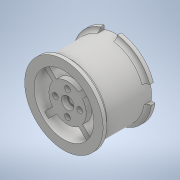
# Autodesk Inventor part: Wheel
Saved by Autodesk Inventor 2020 (Build 240168000, 168)
## iProperties
Created: 2019-03-25
Part Number: Wheel
Material: Типовые
Document SubType Name: Modeling
Designer: cosko
Density: 1 g/cm^3
Appearance: По умолчанию
Mass: 16.7421 g
Surface Area: 120.92 cm^2
Volume: 16.7421 cm^3
Author: cosko
Autodesk Inventor part; units mm, degrees
ref_plane "YZ Plane" through (0, 0, 0) normal (1, 0, 0) x (0, 1, 0)
ref_plane "XZ Plane" through (0, 0, 0) normal (0, 1, 0) x (-1, 0, 0)
ref_plane "XY Plane" through (0, 0, 0) normal (0, 0, 1) x (1, 0, 0)
sketch "Эскиз1" plane through (0, 0, 0) normal (0, 0, 1) x (1, 0, 0)
  line L0 (0, 0) -> (16, 0) construction
  line L1 (16, 0) -> (16, 12) construction
  line L2 (16, 12) -> (16, -16)
  line L3 (16, 12) -> (21, 12)
  line L4 (21, 12) -> (21, -16)
  line L5 (21, -16) -> (16, -16)
  line L6 (16, -16) -> (16, 12)
  line L7 (21, 12) -> (16, 12) construction
  line L8 (16, 12) -> (16, 10) construction
  line L9 (21, 10) -> (21, 10) construction
  line L10 (21, 10) -> (21, 12) construction
  line L11 (21, -16) -> (16, -16) construction
  line L12 (16, -16) -> (16, -14) construction
  line L13 (16, -14) -> (21, -14) construction
  line L14 (21, -14) -> (21, -16) construction
  line L15 (21, -14) -> (21, -14)
  line L16 (19, -12) -> (19, 8)
  line L17 (21, 6) -> (21, -14)
  arc A0 (21, 10) -> (19, 8) centre (21, 8) ccw
  arc A1 (19, -12) -> (21, -14) centre (21, -12) ccw
  arc A2 (21, 10) -> (19, 8) centre (21, 8) ccw
  line L18 (19, 8) -> (19, -12)
  arc A3 (19, -12) -> (21, -14) centre (21, -12) ccw
  line L19 (21, -14) -> (21, 10)
  line L20 (0, 0) -> (0, 12)
  dimension "d0" = 16
  dimension "d1" = 12
  dimension "d2" = 28
  dimension "d3" = 5
  dimension "d4" = 2
  dimension "d7" = 2
  dimension "d46" = 2
  dimension "d47" = 0
  constraints: 42 end point, 8 point on circle, 8 tangent, 7 parallel, 5 horizontal, 4 centre point, 4 perpendicular, 3 point on line, 3 vertical, 1 collinear, 1 equal radius
  measures "d0" distance of L0.start L0.end
  measures "d1" distance of L0.end L1.end
  measures "d2" distance of L1.end L2.end
  measures "d3" distance of L4.end L5.end
  measures "d4" distance of L8.end L7.end
  measures "d7" radius of A0
  measures "d46" distance from line of L13 L2.end
  measures "d47" distance from line of L2.end L5
revolve "Вращение1" add sketch "Эскиз1" angle 360 about axis through (0, 0, 0) along (0, 1, 0) contours L3 L4 A0 L16 A1 L5 L2
sketch "Эскиз2" plane through (0, -16, 0) normal (0, -1, 0) x (1, 0, 0)
  circle A0 centre (0, 0) radius 10
  circle A1 centre (0, 0) radius 2.5
  line L0 (0, 0) -> (0, -5) construction
  line L1 (0, -5) -> (0, 5) construction
  line L2 (0, 5) -> (0, 8) construction
  circle A2 centre (0, 6.5) radius 1.5
  circle A3 centre (-6.5, 0) radius 1.5
  circle A4 centre (0, -6.5) radius 1.5
  circle A5 centre (6.5, 0) radius 1.5
  point P0 (-8, 0)
  point P1 (0, -8)
  point P2 (8, 0)
  dimension "d9" = 20
  dimension "d10" = 5
  dimension "d13" = 3
  dimension "d16" = 360
  dimension "d60" = 13
  constraints: 6 end point, 2 centre point, 2 coincident, 2 horizontal alignment, 2 vertical, 2 vertical alignment, 1 midpoint, 1 point on line, 21 other
  measures "d9" diameter of A0
  measures "d10" diameter of A1
  measures "d13" distance of L1.end L2.end
  measures "d60" distance of point (0, -6.5) point (0, 6.5)
extrude "Выдавливание1" add sketch "Эскиз2" against normal blind 5
sketch "Эскиз3" plane through (0, -16, 0) normal (0, -1, 0) x (1, 0, 0)
  circle A0 centre (0, 0) radius 10 construction
  circle A1 centre (0, 0) radius 16 construction
  circle A2 centre (0, 0) radius 2.5
  line L0 (0, 0) -> (11.3137, -11.3137)
  line L1 (0, 0) -> (16, 0) construction
  line L2 (11.3137, -11.3137) -> (-11.3137, 11.3137)
  line L3 (0, 0) -> (-11.3137, -11.3137)
  line L4 (11.3137, 11.3137) -> (0, 0)
  line L5 (10.253, -12.3744) -> (-1.0607, -1.0607)
  line L6 (-1.0607, -1.0607) -> (1.0607, 1.0607)
  line L7 (1.0607, 1.0607) -> (12.3744, -10.253)
  line L8 (12.3744, -10.253) -> (10.253, -12.3744)
  line L9 (10.253, -12.3744) -> (1.0607, 1.0607) construction
  line L10 (-1.0607, -1.0607) -> (12.3744, -10.253) construction
  line L11 (-12.3744, 10.253) -> (-1.0607, -1.0607)
  line L12 (-1.0607, -1.0607) -> (1.0607, 1.0607)
  line L13 (1.0607, 1.0607) -> (-10.253, 12.3744)
  line L14 (-10.253, 12.3744) -> (-12.3744, 10.253)
  line L15 (-12.3744, 10.253) -> (1.0607, 1.0607) construction
  line L16 (-1.0607, -1.0607) -> (-10.253, 12.3744) construction
  line L17 (12.3744, 10.253) -> (1.0607, -1.0607)
  line L18 (1.0607, -1.0607) -> (-1.0607, 1.0607)
  line L19 (-1.0607, 1.0607) -> (10.253, 12.3744)
  line L20 (10.253, 12.3744) -> (12.3744, 10.253)
  line L21 (12.3744, 10.253) -> (-1.0607, 1.0607) construction
  line L22 (1.0607, -1.0607) -> (10.253, 12.3744) construction
  line L23 (-10.253, -12.3744) -> (1.0607, -1.0607)
  line L24 (1.0607, -1.0607) -> (-1.0607, 1.0607)
  line L25 (-1.0607, 1.0607) -> (-12.3744, -10.253)
  line L26 (-12.3744, -10.253) -> (-10.253, -12.3744)
  line L27 (-10.253, -12.3744) -> (-1.0607, 1.0607) construction
  line L28 (1.0607, -1.0607) -> (-12.3744, -10.253) construction
  circle A3 centre (0, 0) radius 3.25
  circle A4 centre (0, 0) radius 4.5
  point P0 (5.6569, -5.6569)
  point P1 (-5.6569, 5.6569)
  point P2 (5.6569, 5.6569)
  point P3 (-5.6569, -5.6569)
  point P4 (2.4749, -0.3536)
  point P5 (0.3536, -2.4749)
  point P6 (-2.4749, 0.3536)
  point P7 (-0.3536, 2.4749)
  point P8 (0.3536, 2.4749)
  point P9 (2.4749, 0.3536)
  point P10 (-0.3536, -2.4749)
  point P11 (-2.4749, -0.3536)
  dimension "d48" = 45
  dimension "d49" = 3
  dimension "d50" = 3
  dimension "d55" = 6.5
  dimension "d56" = 9
  constraints: 58 end point, 11 parallel, 10 midpoint, 7 perpendicular, 4 point on circle, 4 point on line, 3 centre point, 3 coincident, 1 equal length, 1 horizontal
  measures "d48" angle of L0 L1
  measures "d49" distance of L5.end L6.end
  measures "d50" distance of L17.end L18.end
  measures "d55" diameter of A3
  measures "d56" diameter of A4
sketch "Эскиз4" plane through (0, -11, 0) normal (0, 1, 0) x (1, 0, 0)
  circle A0 centre (0, 0) radius 2.5
  circle A1 centre (0, 0) radius 4
  dimension "d25" = 8
  constraints: 2 centre point, 2 coincident
  measures "d25" diameter of A1
extrude "Выдавливание2" add sketch "Эскиз4" along normal up to surface (23 mm away)
extrude "Выдавливание3" add sketch "Эскиз3" against normal blind 28 contours A2 L4 A3 L17 | L7 A3 L0 A2 | A2 L19 A3 L4 | A3 L4 A4 L17 | L0 A3 L5 A2 | L7 A4 L0 A3 | A3 L19 A4 L4 | A4 L4 L20 L17 | L0 A4 L5 A3 | L7 L8 L0 A4 | A2 L2 A3 L13 | A4 L19 L20 L4 | L23 A3 L3 A2 | L0 L8 L5 A4 | A2 L11 A3 L2 | A3 L2 A4 L13 | L3 A3 L25 A2 | L23 A4 L3 A3 | A3 L11 A4 L2 | A4 L2 L14 L13 | L3 A4 L25 A3 | L23 L26 L3 A4 | A4 L11 L14 L2 | L3 L26 L25 A4
sketch "Эскиз8" plane through (0, 12, 0) normal (0, 1, 0) x (1, 0, 0)
  circle A0 centre (0, 0) radius 19 projected
  circle A1 centre (0, 0) radius 19 projected
  line L0 (2.6463, -18.8148) -> (2.6463, -26.4011)
  line L1 (2.6463, -26.4011) -> (-6.7686, -25.9542)
  line L2 (-6.7686, -25.9542) -> (-6.386, -17.8947)
  circle A2 centre (0, 0) radius 19 projected
  arc A3 (-6.386, -17.8947) -> (2.6463, -18.8148) centre (0, 0) ccw
  line L3 (18.8148, 2.6463) -> (26.4011, 2.6463)
  line L4 (26.4011, 2.6463) -> (25.9542, -6.7686)
  line L5 (25.9542, -6.7686) -> (17.8947, -6.386)
  arc A4 (17.8947, -6.386) -> (18.8148, 2.6463) centre (0, 0) ccw
  line L6 (-2.6463, 18.8148) -> (-2.6463, 26.4011)
  line L7 (-2.6463, 26.4011) -> (6.7686, 25.9542)
  line L8 (6.7686, 25.9542) -> (6.386, 17.8947)
  arc A5 (6.386, 17.8947) -> (-2.6463, 18.8148) centre (0, 0) ccw
  line L9 (-18.8148, -2.6463) -> (-26.4011, -2.6463)
  line L10 (-26.4011, -2.6463) -> (-25.9542, 6.7686)
  line L11 (-25.9542, 6.7686) -> (-17.8947, 6.386)
  arc A6 (-17.8947, 6.386) -> (-18.8148, -2.6463) centre (0, 0) ccw
  dimension "d42" = 360
  constraints: 24 end point, 9 point on circle, 4 centre point, 1 concentric, 1 perpendicular, 1 vertical, 39 other
extrude "Выдавливание5" cut sketch "Эскиз8" against normal blind 10 contours A0 L3 L4 L5 | A0 L6 L7 L8 | L0 L1 L2 A0 | A0 L9 L10 L11
sketch "Эскиз9" plane through (0, 12, 0) normal (0, 1, 0) x (1, 0, 0)
  circle A0 centre (0, 0) radius 2.5
  arc A1 (8.0517, -5.9304) -> (8.0517, 5.9304) centre (0, 0) ccw projected
  arc A2 (-5.9304, -8.0517) -> (5.9304, -8.0517) centre (0, 0) ccw projected
  arc A3 (-8.0517, 5.9304) -> (-8.0517, -5.9304) centre (0, 0) ccw projected
  line L0 (-3.6827, -1.5614) -> (-12.3245, -10.2032) projected
  arc A4 (-3.6827, 1.5614) -> (-3.6827, -1.5614) centre (0, 0) ccw projected
  line L1 (-12.3245, 10.2032) -> (-3.6827, 1.5614) projected
  line L2 (1.5614, 3.6827) -> (5.9304, 8.0517) projected
  arc A5 (5.9304, 8.0517) -> (-5.9304, 8.0517) centre (0, 0) ccw projected
  line L3 (-5.9304, 8.0517) -> (-1.5614, 3.6827) projected
  arc A6 (-1.5614, 3.6827) -> (1.5614, 3.6827) centre (0, 0) ccw projected
  circle A7 centre (6.5, 0) radius 1.5 projected
  line L4 (3.6827, -1.5614) -> (8.0517, -5.9304) projected
  arc A8 (8.0517, -5.9304) -> (8.0517, 5.9304) centre (0, 0) ccw projected
  line L5 (8.0517, 5.9304) -> (3.6827, 1.5614) projected
  arc A9 (3.6827, -1.5614) -> (3.6827, 1.5614) centre (0, 0) ccw projected
  line L6 (5.9304, -8.0517) -> (1.5614, -3.6827) projected
  arc A10 (-1.5614, -3.6827) -> (1.5614, -3.6827) centre (0, 0) ccw projected
  line L7 (-1.5614, -3.6827) -> (-5.9304, -8.0517) projected
  arc A11 (-5.9304, -8.0517) -> (5.9304, -8.0517) centre (0, 0) ccw projected
  circle A12 centre (0, -6.5) radius 1.5 projected
  circle A13 centre (-6.5, 0) radius 1.5 projected
  line L8 (-8.0517, -5.9304) -> (-3.6827, -1.5614) projected
  arc A14 (-3.6827, 1.5614) -> (-3.6827, -1.5614) centre (0, 0) ccw projected
  line L9 (-3.6827, 1.5614) -> (-8.0517, 5.9304) projected
  arc A15 (-8.0517, 5.9304) -> (-8.0517, -5.9304) centre (0, 0) ccw projected
  circle A16 centre (0, 0) radius 11
  circle A17 centre (-8, 0) radius 1.5
  circle A18 centre (8, 0) radius 1.5
  circle A19 centre (0, -8) radius 1.5
  circle A20 centre (0, 8) radius 1.5
  point P0 (-5.9304, -8.0517)
  point P1 (-7.25, 1.299)
  point P2 (-7.25, -1.299)
  point P3 (1.299, -7.25)
  point P4 (-1.299, -7.25)
  point P5 (-1.5614, -3.6827)
  point P6 (-8.7662, -6.6449)
  point P7 (-8.7662, 6.6449)
  dimension "d63" = 22
  dimension "d64" = 3
  dimension "d65" = 3
  dimension "d66" = 16
  dimension "d67" = 8
  dimension "d68" = 3
  dimension "d69" = 3
  dimension "d70" = 16
  dimension "d71" = 8
  constraints: 8 centre point, 1 coincident
  measures "d63" diameter of A16
  measures "d64" diameter of A17
  measures "d65" diameter of A18
  measures "d66" distance of A17.centre A18.centre
  measures "d67" distance of A17.centre point (0, 0)
  measures "d68" diameter of A19
  measures "d69" diameter of A20
  measures "d70" distance of A19.centre A20.centre
  measures "d71" distance of point (0, 0) A19.centre
extrude "Выдавливание6" add sketch "Эскиз9" against normal blind 3 contours L4 A6 L5 A1 | A1 L5 A6 L2 A5 L3 L1 A16 L0 L7 A2 L6 L4 | A6 A4 L3 A5 L2 | L6 A2 L7 A6 | L0 A3 L1 A4 | A18 A7 | A12 A19 | A13 A17 picked at (5.511, 0.058) picked at (-0.0754, -5.511) picked at (-5.5135, -0.1153)
sketch "Эскиз11" plane through (-20.8326, 12, 2.6463) normal (0, 1, 0) x (1, 0, 0)
  circle A0 centre (20.8326, 2.6463) radius 3.5
  dimension "d57" = 7
  constraints: 1 centre point, 1 coincident
  measures "d57" diameter of A0
extrude "Выдавливание8" cut sketch "Эскиз11" against normal blind 3
sketch "Эскиз12" plane through (0, -16, 0) normal (0, -1, 0) x (1, 0, 0)
  circle A0 centre (0, 0) radius 16
  constraints: 1 centre point, 1 coincident
extrude "Выдавливание9" cut sketch "Эскиз12" against normal blind 2
sketch "Эскиз13" plane through (0, -14, 0) normal (0, -1, 0) x (1, 0, 0)
  circle A0 centre (0, 0) radius 3.25
  dimension "d72" = 6.5
  constraints: 1 centre point, 1 coincident
  measures "d72" diameter of A0
extrude "Выдавливание10" cut sketch "Эскиз13" against normal blind 3
